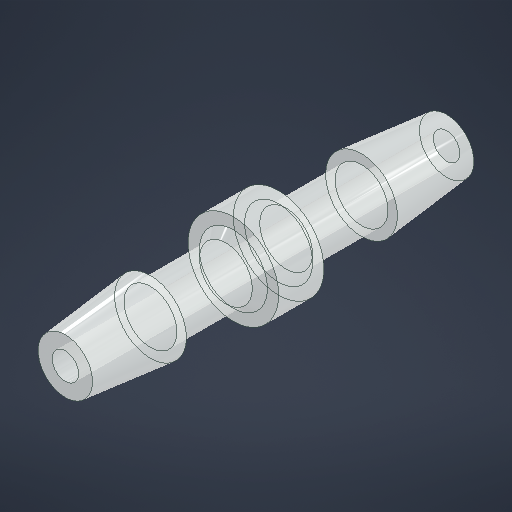
# Autodesk Inventor part: Adafruit_4764
Saved by Autodesk Inventor 2026.2 (Build 302298000, 298)
## iProperties
Created: 2026-02-11
Part Number: Adafruit_4764
Material: Generic
Document SubType Name: Modeling
Designer: vckot
Density: 1 g/cm^3
Appearance: Clear
Author: vckot
Autodesk Inventor part; units mm, degrees
ref_plane "YZ Plane" through (0, 0, 0) normal (1, 0, 0) x (0, 1, 0)
ref_plane "XZ Plane" through (0, 0, 0) normal (0, 1, 0) x (-1, 0, 0)
ref_plane "XY Plane" through (0, 0, 0) normal (0, 0, 1) x (1, 0, 0)
sketch "Sketch1" plane through (0, 0, 0) normal (1, 0, 0) x (0, 1, 0)
  line L0 (0, 12.65) -> (0, -12.65) construction
  line L1 (3, 0) -> (3, 1.5)
  line L2 (3, 1.5) -> (2.25, 1.5)
  line L3 (1.75, 2) -> (1.75, 7)
  line L4 (1.75, 7) -> (2.375, 7)
  line L5 (2.375, 7) -> (1.8, 12.65)
  line L6 (1.8, 12.65) -> (0.875, 12.65)
  line L7 (0.875, 12.65) -> (0.875, 0)
  line L8 (3, 0) -> (-3, 0) construction
  line L9 (3, 0) -> (3, -1.5)
  line L10 (3, -1.5) -> (2.25, -1.5)
  line L11 (1.75, -2) -> (1.75, -7)
  line L12 (1.75, -7) -> (2.375, -7)
  line L13 (2.375, -7) -> (1.8, -12.65)
  line L14 (1.8, -12.65) -> (0.875, -12.65)
  line L15 (0.875, -12.65) -> (0.875, 0)
  line L16 (2.25, 1.5) -> (1.75, 2)
  line L17 (2.25, -1.5) -> (1.75, -2)
  point P0 (0, 0)
  point P1 (1.75, 1.5)
  point P2 (1.75, -1.5)
  dimension "d0" = 25.3
  dimension "d1" = 3
  dimension "d2" = 1.5
  dimension "d3" = 6
  dimension "d4" = 3.5
  dimension "d5" = 5.5
  dimension "d6" = 4.75
  dimension "d7" = 3.6
  dimension "d8" = 1.75
  dimension "d9" = 6
  dimension "d10" = 0.5
  dimension "d11" = 0.5
  dimension "d12" = 0.5
  dimension "d13" = 0.5
  constraints: 36 end point, 6 symmetric about line, 4 point on line, 3 horizontal, 2 vertical, 1 horizontal alignment, 1 midpoint, 1 parallel, 1 perpendicular
  measures "d0" distance of L0.start L0.end
  measures "d1" distance of point (0, 0) L1.start
  measures "d2" distance of L1.start L1.end
  measures "d3" diameter of L1 L0
  measures "d4" diameter of L3 L0
  measures "d5" distance of point (1.75, 1.5) L3.end
  measures "d6" diameter of L4.end L0
  measures "d7" diameter of L5.end L0
  measures "d8" diameter of L7 L0
  measures "d9" distance of L1.start L8.end
  measures "d10" distance of L2.end point (1.75, 1.5)
  measures "d11" distance of L3.start point (1.75, 1.5)
  measures "d12" distance of L10.end point (1.75, -1.5)
  measures "d13" distance of L11.start point (1.75, -1.5)
revolve "Revolution1" add sketch "Sketch1" angle 360 about axis through (0, 0, 12.65) along (0, 0, -1)
equation "\"d11\" = d10"
equation "\"d13\" = d12"
body "Solid1"
